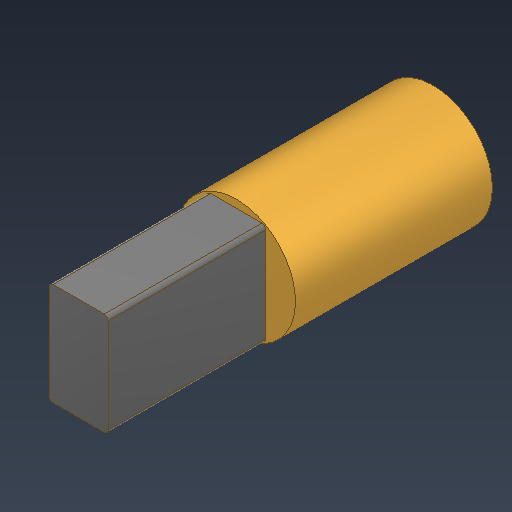
# Autodesk Inventor part: FU650AD5-C6
Saved by Autodesk Inventor 2021 (Build 250183000, 183)
## iProperties
Created: 2021-08-08
Part Number: FU650AD5-C6
Material: ABS プラスチック
Document SubType Name: Modeling
Designer: yuta0
Density: 1.06 g/cm^3
Appearance: 真鍮 - サテン
Mass: 0.428416 g
Surface Area: 3.86002 cm^2
Volume: 0.404166 cm^3
在庫数: 0.0
Author: yuta0
Autodesk Inventor part; units mm, degrees
ref_plane "YZ Plane" through (0, 0, 0) normal (1, 0, 0) x (0, 1, 0)
ref_plane "XZ Plane" through (0, 0, 0) normal (0, 1, 0) x (-1, 0, 0)
ref_plane "XY Plane" through (0, 0, 0) normal (0, 0, 1) x (1, 0, 0)
sketch "スケッチ1" plane through (0, 0, 0) normal (0, 0, 1) x (1, 0, 0)
  circle A0 centre (0, 0) radius 3
  dimension "d0" = 6
  constraints: 1 centre point, 1 coincident
  measures "d0" diameter of A0
extrude "押し出し1" add sketch "スケッチ1" along normal blind 10
sketch "スケッチ2" plane through (0, 0, 0) normal (0, 0, -1) x (-1, 0, 0)
  circle A0 centre (0, 0) radius 1.5
  dimension "d3" = 3
  constraints: 1 centre point, 1 coincident
  measures "d3" diameter of A0
extrude "押し出し2" cut sketch "スケッチ2" against normal blind 1
sketch "スケッチ3" plane through (0, 0, 0) normal (1, 0, 0) x (0, 1, 0)
  line L0 (-3, 0) -> (-3, 10) projected
  line L1 (-3, 10) -> (3, 10) projected
  line L2 (3, 10) -> (3, 0) projected
  line L3 (3, 0) -> (1.5, 0) projected
  line L4 (1.5, 0) -> (1.5, 1) projected
  line L5 (1.5, 1) -> (-1.5, 1) projected
  line L6 (-1.5, 1) -> (-1.5, 0) projected
  line L7 (-1.5, 0) -> (-3, 0) projected
  arc A0 (-1.5, 1) -> (1.5, 1) centre (0, 1.625) ccw
  line L8 (0, 0) -> (0, 1)
  constraints: 3 point on circle, 2 end point, 1 centre point, 1 coincident, 1 midpoint
revolve "回転1" add sketch "スケッチ3" angle 360 about axis through (0, 0, 0) along (0, 0, 1) picked at (0.9377, 0.8892) contours L5 A0 L8
sketch "スケッチ4" plane through (0, 0, 10) normal (0, 0, 1) x (1, 0, 0)
  circle A0 centre (0, 0) radius 3 projected
  line L0 (1.5, 2.5981) -> (-1.5, 2.5981)
  line L1 (-1.5, 2.5981) -> (-1.5, -2.5981)
  line L2 (-1.5, -2.5981) -> (1.5, -2.5981)
  line L3 (1.5, -2.5981) -> (1.5, 2.5981)
  line L4 (1.5, 2.5981) -> (-1.5, -2.5981) construction
  line L5 (-1.5, 2.5981) -> (1.5, -2.5981) construction
  dimension "d7" = 3
  constraints: 12 end point, 2 midpoint, 2 parallel, 1 horizontal, 1 perpendicular, 2 other
  measures "d7" distance of L1.end L2.end
extrude "押し出し3" add sketch "スケッチ4" along normal blind 8 contours L3 L2 L1 L0
fillet "フィレット1" radius 0.2 4 edges at (-1.5, -2.5981, 14) (1.5, -2.5981, 14) (-1.5, 2.5981, 14) (1.5, 2.5981, 14)
